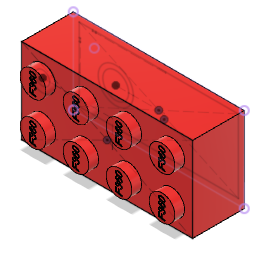
LEGO Parametric v5 (Autodesk Fusion 360 design; units mm, degrees)
Autodesk Fusion 360 part; units mm, degrees
note: some values were not read from the file. Chosen so that the rebuilt part matches the saved one: which bodies a step acts on.
sketch "Top" plane through (0, 0, 0) normal (0, 0, 1) x (1, 0, 0) in component "LEGO"
  line L0 (15.9, 7.9) -> (-15.9, 7.9)
  line L1 (-15.9, 7.9) -> (-15.9, -7.9)
  line L2 (-15.9, -7.9) -> (15.9, -7.9)
  line L3 (15.9, -7.9) -> (15.9, 7.9)
  line L4 (15.9, 7.9) -> (-15.9, -7.9) construction
  line L5 (-15.9, 7.9) -> (15.9, -7.9) construction
  line L6 (0, 0) -> (1, 0) construction
  line L7 (1, 0) -> (1, -1) construction
  line L8 (1, -1) -> (1, 4) construction
  line L9 (1, 4) -> (-12, 4) construction
  circle A0 centre (-12, 4) radius 2.4
  circle A1 centre (-12, 4) radius 1.3
  dimension "d7" = 31.8
  dimension "d8" = 15.8
  dimension "d12" = 1
  dimension "d13" = 1
  dimension "d14" = 5
  dimension "d15" = 13
  dimension "d27" = 4.8
  dimension "d29" = 2.6
  constraint horizontal L0
  constraint perpendicular L0 L1
  constraint parallel L0 L2
  constraint parallel L1 L3
  constraint coincident L4 L6.start
  constraint coincident L5 L6.start
  constraint coincident L6.start origin
  constraint horizontal L6
  constraint perpendicular L6 L7
  constraint perpendicular L2 L8
  constraint perpendicular L8 L9
  constraint coincident L9.end A0.centre
  constraint concentric A0 A1
  measures "d7" distance of L1.end L2.end
  measures "d8" distance of L0.end L1.end
  measures "d12" distance of L6.start L6.end
  measures "d13" distance of L6.end L7.end
  measures "d14" distance of L7.end L8.end
  measures "d15" distance of L8.end L9.end
  measures "d27" diameter of A0
  measures "d29" diameter of A1
ref_plane "WorkPlane1" through (0, 0, -9.6) normal (0, 0, 1) x (1, 0, 0) in component "LEGO"
ref_plane "WorkPlane2" through (0, 0, -1) normal (0, 0, 1) x (1, 0, 0) in component "LEGO"
sketch "Bottom" plane through (0, 0, -9.6) normal (0, 0, 1) x (1, 0, 0) in component "LEGO"
  line L0 (-15.9, -7.9) -> (15.9, -7.9)
  line L1 (-15.9, 7.9) -> (-15.9, -7.9)
  line L2 (15.9, 7.9) -> (-15.9, 7.9)
  line L3 (15.9, -7.9) -> (15.9, 7.9)
  line L4 (14.8, 6.8) -> (-14.8, 6.8)
  line L5 (-14.8, 6.8) -> (-14.8, -6.8)
  line L6 (-14.8, -6.8) -> (14.8, -6.8)
  line L7 (14.8, -6.8) -> (14.8, 6.8)
  line L8 (14.8, 6.8) -> (-14.8, -6.8) construction
  line L9 (-14.8, 6.8) -> (14.8, -6.8) construction
  line L10 (1, -1) -> (1, 0) construction
  line L11 (1, 0) -> (-8, 0) construction
  circle A0 centre (-8, 0) radius 2.4
  circle A1 centre (-8, 0) radius 3.2569
  line L12 (0, 6.8) -> (1.3, 6.8) construction
  line L13 (1.3, 6.8) -> (1.3, 6.6) construction
  line L14 (1.3, 6.6) -> (-11.7, 6.6) construction
  line L15 (-11.7, 6.6) -> (-11.7, 6.8)
  line L16 (-11.7, 6.6) -> (-12.3, 6.6)
  line L17 (-12.3, 6.6) -> (-12.3, 6.8)
  line L18 (-14.8, 0) -> (-14.8, -1.3) construction
  line L19 (-14.8, -1.3) -> (-14.6, -1.3) construction
  line L20 (-14.6, -1.3) -> (-14.6, 3.7) construction
  line L21 (-14.6, 3.7) -> (-14.8, 3.7)
  line L22 (-14.6, 3.7) -> (-14.6, 4.3)
  line L23 (-14.6, 4.3) -> (-14.8, 4.3)
  point P0 (-12, 4)
  point P1 (1, -1)
  dimension "d19" = 29.6
  dimension "d20" = 13.6
  dimension "d23" = 1
  dimension "d24" = 9
  dimension "d25" = 4.8
  dimension "d26" = 6.5137
  dimension "d31" = 1.3
  dimension "d32" = 0.2
  dimension "d33" = 13
  dimension "d34" = 0.6
  dimension "d35" = 1.3
  dimension "d36" = 0.2
  dimension "d37" = 5
  dimension "d38" = 0.6
  constraint horizontal L4
  constraint perpendicular L4 L5
  constraint parallel L4 L6
  constraint parallel L5 L7
  constraint coincident L8 origin
  constraint coincident L9 origin
  constraint coincident P1 L10.start
  constraint vertical L10
  constraint perpendicular L10 L11
  constraint coincident L11.end A0.centre
  constraint concentric A0 A1
  constraint midpoint L4 L12.start
  constraint horizontal L12
  constraint perpendicular L12 L13
  constraint perpendicular L13 L14
  constraint coincident L4 L15.end
  constraint perpendicular L4 L15
  constraint perpendicular L15 L16
  constraint coincident L4 L17.end
  constraint perpendicular L4 L17
  constraint midpoint L5 L18.start
  constraint parallel L5 L18
  constraint perpendicular L5 L19
  constraint perpendicular L19 L20
  constraint coincident L5 L21.end
  constraint perpendicular L5 L21
  constraint perpendicular L21 L22
  constraint coincident L5 L23.end
  constraint perpendicular L5 L23
  measures "d19" distance of L5.end L6.end
  measures "d20" distance of L4.end L5.end
  measures "d23" distance of P1 L10.end
  measures "d24" distance of L10.end L11.end
  measures "d25" diameter of A0
  measures "d26" diameter of A1
  measures "d31" distance of L12.start L12.end
  measures "d32" distance of L12.end L13.end
  measures "d33" distance of L13.end L14.end
  measures "d34" distance of L14.end L16.end
  measures "d35" distance of L18.start L18.end
  measures "d36" distance of L18.end L19.end
  measures "d37" distance of L19.end L20.end
  measures "d38" distance of L20.end L22.end
ref_plane "WorkPlane3" through (0, 0, 1.8) normal (0, 0, 1) x (1, 0, 0) in component "LEGO"
sketch "PegTop" plane through (0, 0, 1.8) normal (0, 0, 1) x (1, 0, 0) in component "LEGO"
  circle A0 centre (-12, 4) radius 2.4
sketch "Underside of top" plane through (0, 0, -1) normal (0, 0, 1) x (1, 0, 0) in component "LEGO"
  circle A0 centre (-12, 4) radius 1.3
  line L0 (14.8, 6.8) -> (-14.8, 6.8)
  line L1 (14.8, -6.8) -> (14.8, 6.8)
  line L2 (-14.8, -6.8) -> (14.8, -6.8)
  line L3 (-14.8, 6.8) -> (-14.8, -6.8)
  circle A1 centre (-8, 0) radius 3.2569
  circle A2 centre (-8, 0) radius 2.4
  line L4 (-11.7, 6.6) -> (-11.7, 6.8)
  line L5 (-11.7, 6.6) -> (-12.3, 6.6)
  line L6 (-12.3, 6.6) -> (-12.3, 6.8)
  line L7 (-14.6, 4.3) -> (-14.8, 4.3)
  line L8 (-14.6, 3.7) -> (-14.6, 4.3)
  line L9 (-14.6, 3.7) -> (-14.8, 3.7)
ref_plane "WorkPlane4" through (0, 0, 0.7) normal (0, 0, 1) x (1, 0, 0) in component "LEGO"
sketch "Inside of peg" plane through (0, 0, 0.7) normal (0, 0, 1) x (1, 0, 0) in component "LEGO"
  circle A0 centre (-12, 4) radius 1.3
extrude "Extrude1" add sketch "Bottom" along normal blind 9.6 contours L0 L1 L2 L3 makes body 1 in component "LEGO"
extrude "Extrude2" add sketch "Top" against normal blind 1 contours L0 L1 L2 L3 | A0 | A1 bodies 1 in component "LEGO"
loft "Loft1" add profiles "Underside of top", "Inside of peg" section 1 contours A0 section 2 separate body makes body 2 in component "LEGO"
loft "Loft2" add profiles "PegTop", "Top" section 1 section 2 contours A0 | A1 separate body makes body 3 in component "LEGO"
extrude "Extrude1'" add sketch "Bottom" along normal up to surface (8.6 mm away) separate body contours A1 makes body 4 in component "Component"
extrude "Extrude3" add sketch "Bottom" along normal up to surface (8.6 mm away) separate body contours L4 L15 L16 L17 | L5 L21 L22 L23 makes body 5 at (-14.8, 4.1, -6.7333) makes body 6 at (-11.9, 6.6, -6.7333) in component "LEGO"
fillet "Fillet1" radius 0.2 2 edges at (-14.6, 4, -9.6) (-12, 6.6, -9.6) on bodies 5 6 in component "LEGO"
pattern_linear "R-Pattern1" count 4 spacing 8 along (1, 0, 0) count 2 spacing 8 along (0, -1, 0) of bodies 3 makes body 7 at (-1.6119, 3.761, 1.2) makes body 8 at (6.3881, 3.761, 1.2) makes body 9 at (14.3881, 3.761, 1.2) makes body 10 at (-9.6119, -4.239, 1.2) makes body 11 at (-1.6119, -4.239, 1.2) makes body 12 at (6.3881, -4.239, 1.2) makes body 13 at (14.3881, -4.239, 1.2) in component "LEGO"
combine "Combine2" operation add target body 1 tool bodies 7 9 11 10 8 12 13 3 in component "LEGO"
pattern_linear "R-Pattern2" count 2 spacing 8 along (0, -1, 0) count 4 spacing 8 along (1, 0, 0) of bodies 2 makes body 14 at (-10.7016, -4.0648, -0.4333) makes body 15 at (-2.7016, 3.9352, -0.4333) makes body 16 at (-2.7016, -4.0648, -0.4333) makes body 17 at (5.2984, 3.9352, -0.4333) makes body 18 at (5.2984, -4.0648, -0.4333) makes body 19 at (13.2984, 3.9352, -0.4333) makes body 20 at (13.2984, -4.0648, -0.4333) in component "LEGO"
combine "Combine1" operation cut target body 1 tool bodies 20 15 16 17 18 19 14 2 in component "LEGO"
sketch "Text" plane through (0, 0, 1.8) normal (0, 0, 1) x (1, 0, 0) in component "LEGO"
  circle A0 centre (-12, -4) radius 2.4
  circle A1 centre (-12, 4) radius 2.4
  line L0 (-11.3791, 2.0998) -> (-11.3827, 5.9014) construction
  line L1 (-11.3827, 5.9014) -> (-12.6209, 5.9002) construction
  line L2 (-12.6209, 5.9002) -> (-12.6173, 2.0986) construction
  line L3 (-12.6173, 2.0986) -> (-11.3791, 2.0998) construction
  line L4 (-11.3809, 4.0006) -> (-12.6191, 3.9994) construction
  point P0 (-12, 4)
  point P1 (-12, 4)
  text T0 "F360" font "Arial" height 1.2 italic align left top in box 3.8016 x 1.2382 at (-11.3791, 2.0998) x (-0.000923, 1) y (-1, -0.000923) spacing 1
  constraint midpoint L0 L4.start
  constraint midpoint L2 L4.end
  constraint perpendicular L2 L4
  constraint midpoint L4 P1
  constraint coincident P1 P0
extrude "Extrude4" add sketch "Text" along normal blind 0.05 separate body text T0 makes body 21 at (-12.0314, 3.7065, 1.8) makes body 22 at (-11.8885, 4.1763, 1.8) makes body 23 at (-11.9825, 5.732, 1.8) makes body 24 at (-11.999, 2.2741, 1.8) in component "LEGO"
pattern_linear "R-Pattern3" count 4 spacing 8 along (1, 0, 0) count 2 spacing 8 along (0, -1, 0) of bodies 21 22 23 24 makes body 25 at (-4.0314, 3.7065, 1.8) makes body 26 at (3.9686, 3.7065, 1.8) makes body 27 at (11.9686, 3.7065, 1.8) makes body 28 at (-12.0314, -4.2935, 1.8) makes body 29 at (-4.0314, -4.2935, 1.8) makes body 30 at (3.9686, -4.2935, 1.8) makes body 31 at (11.9686, -4.2935, 1.8) makes body 32 at (-3.8885, 4.1763, 1.8) makes body 33 at (4.1115, 4.1763, 1.8) makes body 34 at (12.1115, 4.1763, 1.8) makes body 35 at (-11.8885, -3.8237, 1.8) makes body 36 at (-3.8885, -3.8237, 1.8) makes body 37 at (4.1115, -3.8237, 1.8) makes body 38 at (12.1115, -3.8237, 1.8) makes body 39 at (-3.9825, 5.732, 1.8) makes body 40 at (4.0175, 5.732, 1.8) makes body 41 at (12.0175, 5.732, 1.8) makes body 42 at (-11.9825, -2.268, 1.8) makes body 43 at (-3.9825, -2.268, 1.8) makes body 44 at (4.0175, -2.268, 1.8) makes body 45 at (12.0175, -2.268, 1.8) makes body 46 at (-3.999, 2.2741, 1.8) makes body 47 at (4.001, 2.2741, 1.8) makes body 48 at (12.001, 2.2741, 1.8) makes body 49 at (-11.999, -5.7259, 1.8) makes body 50 at (-3.999, -5.7259, 1.8) makes body 51 at (4.001, -5.7259, 1.8) makes body 52 at (12.001, -5.7259, 1.8) in component "LEGO"
combine "Combine3" operation add target body 1 tool bodies 21 36 47 46 41 43 52 51 33 28 40 42 49 50 44 45 32 30 39 38 35 34 48 37 22 23 25 26 27 29 31 24 in component "LEGO"
extrude "Extrude5" add sketch "Bottom" along normal up to surface (8.6 mm away) separate body contours A1 makes body 53 in component "LEGO"
pattern_linear "R-Pattern4" count 3 spacing 8 along (1, 0, 0) of bodies 53 makes body 54 at (3.2528, -0.1623, -3.8667) makes body 55 at (11.2528, -0.1623, -3.8667) in component "LEGO"
pattern_linear "R-Pattern5" count 2 spacing 8 along (0, -1, 0) of bodies 5 makes body 56 in component "LEGO"
pattern_linear "R-Pattern6" count 4 spacing 8 along (1, 0, 0) of bodies 6 makes body 57 at (-3.9, 6.8, -6.7333) makes body 58 at (4.1, 6.8, -6.7333) makes body 59 at (12.1, 6.8, -6.7333) in component "LEGO"
component "LEGO" placed x (1, 0, 0) y (0, 1, 0) z (0, 0, 1) at (0, 0, 0)
component "Component" placed x (1, 0, 0) y (0, 1, 0) z (0, 0, 1) at (0, 0, 0) in component "LEGO"
equation "BrickLen = 4" comment "Lengh, in lego studs"
equation "BrickWid = 2" comment "Width, in lego studs"
equation "BrickHt = 3" comment "Height, in lego plate-thickness units (3 is a standard brick height)"
equation "LU = 1.6 mm" comment "This is the standard lego size unit, which everythign scales from. It's never used direclty (always has gaps added)"
equation "OuterWallGap = LU / 16" comment "Must have spacing, otherwise nothing fits"
equation "StudGap = LU / 32" comment "Adjust this to adjust fit snugness (bigger numbers = looser fits) - this is not a LEGO unit - it's for you to adjust to suit your printer"
equation "d7 = BrickLen * 5 * LU - 2 * OuterWallGap"
equation "d8 = BrickWid * 5 * LU - 2 * OuterWallGap"
equation "TopGap = LU / 50 * 0" comment "Adjust this if your 3D printer tolerance gets heights wrong (add to here to shrink the height)"
equation "d12 = One"
equation "d13 = One"
equation "d14 = ( BrickWid - 1 ) * 5 * LU / 2 + One"
equation "d15 = ( BrickLen - 1 ) * 5 * LU / 2 + One"
equation "One = LU / 1.6" comment "Cannot have parametrics lengths of 0, so we add one to things that might become zero..."
equation "d17 = -BrickHt * 2 * LU - 2 * TopGap"
equation "d18 = -1 * 5 / 8 * LU + TopGap"
equation "d19 = BrickLen * 5 * LU - 2 * OuterWallThickness"
equation "d20 = BrickWid * 5 * LU - 2 * OuterWallThickness"
equation "OuterWallThickness = LU * 3 / 4" comment "Don't change"
equation "StudNub = LU / 8" comment "Adjust this to adjust fit snugness (bigger numbers = looser fits) - this is the little bar inside the brick"
equation "d23 = ( BrickWid - 2 ) * 5 * LU / 2 + One"
equation "d24 = ( BrickLen - 2 ) * 5 * LU / 2 + One"
equation "d25 = 3 * LU"
equation "d26 = LU * 5 * 2 ^ 0.5 - LU * 3"
equation "d27 = 3 * LU"
equation "d28 = LU + 2 * OuterWallGap"
equation "d29 = 13 / 8 * LU"
equation "d30 = LU + OuterWallGap"
equation "d31 = One + LU * 3 / 8 / 2"
equation "d32 = LU / 8"
equation "d33 = ( BrickLen - 1 ) * 5 * LU / 2 + One"
equation "d34 = LU * 3 / 8"
equation "d35 = One + LU * 3 / 8 / 2"
equation "d36 = LU / 8"
equation "d37 = ( BrickWid - 1 ) * 5 * LU / 2 + One"
equation "d38 = LU * 3 / 8"
equation "d39 = BrickHt * 2 * LU - 2 * TopGap"
equation "d41 = -1 * 5 / 8 * LU + TopGap"
equation "d48 = LU / 8"
equation "d49 = BrickLen"
equation "d50 = BrickWid"
equation "d51 = LU * 5"
equation "d52 = -LU * 5"
equation "d53 = BrickWid"
equation "d54 = BrickLen"
equation "d55 = -LU * 5"
equation "d56 = LU * 5"
equation "d57 = LU / 16 / 2"
equation "d59 = BrickLen"
equation "d60 = BrickWid"
equation "d61 = LU * 5"
equation "d62 = -LU * 5"
equation "d65 = BrickLen - 1"
equation "d66 = BrickWid - 1"
equation "d67 = LU * 5"
equation "d68 = LU * 5"
equation "d69 = BrickWid"
equation "d71 = -LU * 5"
equation "d73 = BrickLen"
equation "d75 = LU * 5"
named bodies: "Brick", "PegCut", "Peg", "Spacer1", "Spacer2", "Peg (1)", "Peg (2)", "Peg (3)", "Peg (4)", "Peg (5)", "Peg (6)", "Peg (7)", "PegCut (1)", "PegCut (2)", "PegCut (3)", "PegCut (4)", "PegCut (5)", "PegCut (6)", "PegCut (7)", "Gut", "Gut (1)", "Gut (2)", "Spacer1 (1)", "Spacer2 (1)", "Spacer2 (2)", "Spacer2 (3)"
